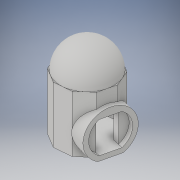
# Autodesk Inventor part: dome one terminal
Saved by Autodesk Inventor 2017 (Build 210142000, 142)
## iProperties
Created: 2018-03-05
Part Number: dome one terminal
Material: Generic
Document SubType Name: Modeling
Designer: Braxton
Density: 1 g/cm^3
Appearance: Default
Author: Braxton
Autodesk Inventor part; units mm, degrees
ref_plane "YZ Plane" through (0, 0, 0) normal (1, 0, 0) x (0, 1, 0)
ref_plane "XZ Plane" through (0, 0, 0) normal (0, 1, 0) x (-1, 0, 0)
ref_plane "XY Plane" through (0, 0, 0) normal (0, 0, 1) x (1, 0, 0)
sketch "Sketch1" plane through (0, 0, 0) normal (0, 1, 0) x (-1, 0, 0)
  line L0 (129.9296, -78.9016) -> (58.7381, -140.2035)
  line L1 (58.7381, -140.2035) -> (-34.8894, -147.9524)
  line L2 (-34.8894, -147.9524) -> (-115.1904, -99.1885)
  line L3 (-115.1904, -99.1885) -> (-151.4925, -12.538)
  line L4 (-151.4925, -12.538) -> (-129.9296, 78.9016)
  line L5 (-129.9296, 78.9016) -> (-58.7381, 140.2035)
  line L6 (-58.7381, 140.2035) -> (34.8894, 147.9524)
  line L7 (34.8894, 147.9524) -> (115.1904, 99.1885)
  line L8 (115.1904, 99.1885) -> (151.4925, 12.538)
  line L9 (151.4925, 12.538) -> (129.9296, -78.9016)
  point P0 (0, 0)
  point P1 (0, 0)
  dimension "d0" = 289.1411
  constraints: 20 end point, 1 coincident, 21 other
  measures "d0" distance between parallel lines of L5 L0
extrude "bace" add sketch "Sketch1" along normal blind 25.4
sketch "Sketch2" plane through (0, 25.4, 0) normal (0, 1, 0) x (1, 0, 0)
  line L0 (-58.7381, 140.2035) -> (-129.9296, 78.9016) projected
  line L1 (-129.9296, 78.9016) -> (-58.7381, 140.2035)
  line L2 (-58.7381, 140.2035) -> (34.8894, 147.9524)
  line L3 (34.8894, 147.9524) -> (115.1904, 99.1885)
  line L4 (115.1904, 99.1885) -> (151.4925, 12.538)
  line L5 (151.4925, 12.538) -> (129.9296, -78.9016)
  line L6 (129.9296, -78.9016) -> (58.7381, -140.2035)
  line L7 (58.7381, -140.2035) -> (-34.8894, -147.9524)
  line L8 (-34.8894, -147.9524) -> (-115.1904, -99.1885)
  line L9 (-115.1904, -99.1885) -> (-151.4925, -12.538)
  line L10 (-151.4925, -12.538) -> (-129.9296, 78.9016)
  line L11 (-107.1019, 65.0392) -> (-48.4182, 115.5708)
  line L12 (-48.4182, 115.5708) -> (28.7596, 121.9582)
  line L13 (28.7596, 121.9582) -> (94.9523, 81.7618)
  line L14 (94.9523, 81.7618) -> (124.8764, 10.3351)
  line L15 (124.8764, 10.3351) -> (107.1019, -65.0392)
  line L16 (107.1019, -65.0392) -> (48.4182, -115.5708)
  line L17 (48.4182, -115.5708) -> (-28.7596, -121.9582)
  line L18 (-28.7596, -121.9582) -> (-94.9523, -81.7618)
  line L19 (-94.9523, -81.7618) -> (-124.8764, -10.3351)
  line L20 (-124.8764, -10.3351) -> (-107.1019, 65.0392)
  line L21 (-129.9296, 78.9016) -> (-151.4925, -12.538) projected
  point P0 (0, 0)
  point P1 (0, 0)
  point P2 (0, 0)
  dimension "d4" = 25.4
  constraints: 40 end point, 2 coincident, 1 parallel, 42 other
  measures "d4" distance between parallel lines of L21 L20
extrude "bace wall" add sketch "Sketch2" along normal blind 254
sketch "Sketch3" plane through (0, 279.4, 0) normal (0, 1, 0) x (1, 0, 0)
  line L0 (-115.1904, -99.1885) -> (-151.4925, -12.538) projected
  circle A0 centre (0, 0) radius 119.1705
  line L1 (-58.7381, 140.2035) -> (-129.9296, 78.9016)
  line L2 (-129.9296, 78.9016) -> (-151.4925, -12.538)
  line L3 (-151.4925, -12.538) -> (-115.1904, -99.1885)
  line L4 (-115.1904, -99.1885) -> (-34.8894, -147.9524)
  line L5 (-34.8894, -147.9524) -> (58.7381, -140.2035)
  line L6 (58.7381, -140.2035) -> (129.9296, -78.9016)
  line L7 (129.9296, -78.9016) -> (151.4925, 12.538)
  line L8 (151.4925, 12.538) -> (115.1904, 99.1885)
  line L9 (115.1904, 99.1885) -> (34.8894, 147.9524)
  line L10 (34.8894, 147.9524) -> (-58.7381, 140.2035)
  line L11 (-129.9296, 78.9016) -> (-58.7381, 140.2035) projected
  line L12 (34.8894, 147.9524) -> (115.1904, 99.1885) projected
  line L13 (115.1904, 99.1885) -> (151.4925, 12.538) projected
  line L14 (151.4925, 12.538) -> (129.9296, -78.9016) projected
  line L15 (-34.8894, -147.9524) -> (58.7381, -140.2035) projected
  line L16 (-124.8764, -10.3351) -> (-107.1019, 65.0392) projected
  point P0 (-115.9892, 27.352)
  constraints: 20 end point, 2 coincident, 1 midpoint, 3 other
extrude "bace cieiling" add sketch "Sketch3" along normal blind 25.4
ref_plane "dome work plane" through (8.8872, 25.4, -37.6872) normal (0.9733039, 0, 0.22952) x (0.22952, 0, -0.9733039)
sketch "Sketch10" plane through (8.8872, 25.4, -37.6872) normal (0.9733039, 0, 0.22952) x (0.22952, 0, -0.9733039)
  line L0 (105.8497, 279.4) -> (80.4497, 279.4)
  line L1 (-157.8914, 279.4) -> (80.4497, 279.4) projected
  arc A0 (80.4497, 279.4) -> (-38.7209, 398.5705) centre (-38.7209, 279.4) ccw
  arc A1 (105.8497, 279.4) -> (-38.7209, 423.9705) centre (-38.7209, 279.4) ccw
  line L2 (-38.7209, 423.9705) -> (-38.7209, 398.5705)
  line L3 (-38.7209, 398.5705) -> (-38.7209, 279.4) construction
  point P0 (-38.7209, -25.4)
  dimension "d32" = 119.1705
  dimension "d33" = 144.5705
  constraints: 6 end point, 4 point on circle, 2 centre point, 2 coincident, 2 vertical, 1 midpoint
  measures "d32" radius of A0
  measures "d33" radius of A1
revolve "dome" add sketch "Sketch10" angle 360 about axis through (0, 423.9705, 0) along (0, -1, 0)
sketch "Sketch8" plane through (151.4925, 0, -12.538) normal (0.9733039, 0, 0.22952) x (0.22952, 0, -0.9733039)
  line L0 (-46.9738, 25.4) -> (3.8262, 25.4)
  line L1 (3.8262, 25.4) -> (3.8262, 194.7333)
  line L2 (3.8262, 194.7333) -> (-46.9738, 194.7333)
  line L3 (-46.9738, 194.7333) -> (-46.9738, 25.4)
  line L4 (-46.9738, 25.4) -> (-97.7738, 25.4)
  line L5 (-97.7738, 25.4) -> (-97.7738, 194.7333)
  line L6 (-97.7738, 194.7333) -> (-46.9738, 194.7333)
  line L7 (-85.6947, 25.4) -> (-8.253, 25.4) projected
  line L8 (-46.9738, 25.4) -> (-46.9738, 0) construction
  dimension "d16" = 50.8
  dimension "d17" = 169.3333
  constraints: 16 end point, 2 collinear, 2 symmetric about line, 1 horizontal, 1 midpoint, 1 perpendicular, 1 vertical
  measures "d16" distance of L0.start L0.end
  measures "d17" distance of L0.end L1.end
extrude "door frame" cut sketch "Sketch8" against normal blind 42.8625
sketch "Sketch7" plane through (151.4925, 0, -12.538) normal (0.9733039, 0, 0.22952) x (0.22952, 0, -0.9733039)
  line L0 (-97.7738, 194.7333) -> (3.8262, 194.7333)
  line L1 (-97.7738, 25.4) -> (3.8262, 25.4)
  arc A0 (10.4321, 0) -> (-104.3797, 0) centre (-46.9738, 110.0667) ccw
  arc A1 (-97.7738, 194.7333) -> (-97.7738, 25.4) centre (-46.9738, 110.0667) ccw
  arc A2 (3.8262, 25.4) -> (3.8262, 194.7333) centre (-46.9738, 110.0667) ccw
  line L2 (-104.3797, 0) -> (10.4321, 0)
  line L3 (-93.9476, 0) -> (-93.9476, 304.8) projected
  line L4 (-93.9476, 194.7333) -> (-93.9476, 224.9734)
  line L5 (-85.6947, 25.4) -> (-148.3463, 25.4) projected
  line L6 (-93.9476, 25.4) -> (-93.9476, 0)
  line L7 (0, 0) -> (0, 304.8) projected
  line L8 (0, 224.9734) -> (0, 194.7333)
  line L9 (0, 25.4) -> (0, 0)
  point P0 (-46.9738, 0)
  point P1 (-46.9738, 0)
  dimension "d14" = 169.3333
  dimension "d15" = 101.6
  dimension "d36" = 25.4
  dimension "d37" = 25.4
  constraints: 14 end point, 12 point on line, 8 point on circle, 3 centre point, 3 coincident, 2 horizontal, 2 parallel, 1 collinear, 1 concentric, 1 midpoint
  measures "d14" distance between parallel lines of L1 L0
  measures "d15" distance of L0.start L0.end
  measures "d36" distance between parallel lines of L2 L1
  measures "d37" radial gap between concentric circles of A0 A1
extrude "corridor connection" add sketch "Sketch7" along normal blind 25.4 contours A1 L5 A0 L3 L0 | L3 A0 L7 L0 | L1 L3 L2 A0 L5 | L7 A0 L2 L1 A2 L0 | L1 L7 L2 L3
sketch "Sketch11" plane through (151.4925, 224.9734, -12.538) normal (0.9733039, 0, 0.22952) x (0.22952, 0, -0.9733039)
  line L0 (76.0052, -224.9734) -> (0, -224.9734) projected
  line L1 (-85.6947, -30.2401) -> (-97.7738, -30.2401) projected
  line L2 (0, -224.9734) -> (0, 79.8266) projected
  line L3 (-93.9476, -30.2401) -> (-93.9476, 0)
  line L4 (0, 0) -> (0, -30.2401)
  line L5 (-93.9476, -224.9734) -> (0, -224.9734) projected
  line L6 (-93.9476, -224.9734) -> (-93.9476, -205.7351)
  line L7 (0, -208.7724) -> (0, -224.9734)
  line L8 (-104.3797, -224.9734) -> (-93.9476, -224.9734)
  line L9 (0, -224.9734) -> (10.4321, -224.9734)
  arc A0 (10.4321, -224.9734) -> (0, 0) centre (-46.9738, -114.9068) ccw
  arc A1 (-93.9476, 0) -> (-104.3797, -224.9734) centre (-46.9738, -114.9068) ccw
  line L10 (-97.7738, -30.2401) -> (-93.9476, -30.2401)
  line L11 (0, -30.2401) -> (3.8262, -30.2401)
  line L12 (-97.7738, -199.5734) -> (-93.9476, -199.5734)
  line L13 (-85.6947, -199.5734) -> (-148.3463, -199.5734) projected
  line L14 (-93.9476, -205.7351) -> (-93.9476, -199.5734)
  line L15 (0, -208.7724) -> (0, -199.5734)
  line L16 (3.8262, -199.5734) -> (0, -199.5734) projected
  line L17 (0, -199.5734) -> (3.8262, -199.5734)
  line L18 (-97.7738, -30.2401) -> (-97.7738, -199.5734) projected
  line L19 (-97.7738, -30.2401) -> (-97.7738, -199.5734)
  line L20 (3.8262, -30.2401) -> (3.8262, -199.5734) projected
  line L21 (3.8262, -30.2401) -> (3.8262, -199.5734)
  arc A2 (0, 0) -> (-93.9476, 0) centre (-46.9738, -114.9068) ccw projected
  arc A3 (-93.9476, 0) -> (-104.3797, -224.9734) centre (-46.9738, -114.9068) ccw projected
  point P0 (-46.9738, -224.9734)
  point P1 (-38.7209, -117.9441)
  point P2 (3.8262, -199.5734)
  constraints: 28 end point, 9 point on line, 4 collinear, 4 point on circle, 2 centre point, 2 concentric, 2 perpendicular, 1 horizontal alignment, 1 vertical
extrude "hide sliding doors" add sketch "Sketch11" against normal up to next contours L0 L2 L16 L20 L11 A0 | L8 A1 L13 L12 L14 L6 | L3 L1 L18 L13 A1
sketch "Sketch9" plane through (104.3295, 25.4, 76.7959) normal (0.22952, 0, -0.9733039) x (-0.9733039, 0, -0.22952)
  line L0 (-12.7, 169.3333) -> (-6.35, 169.3333)
  line L1 (-6.35, 169.3333) -> (-6.35, 0)
  line L2 (-6.35, 0) -> (-19.05, 0)
  line L3 (-19.05, 0) -> (-19.05, 169.3333)
  line L4 (-12.7, 169.3333) -> (-19.05, 169.3333)
  line L5 (-25.4, 199.5734) -> (-25.4, 208.8041) projected
  point P0 (119.1705, -25.4)
  point P1 (-25.4, -25.4)
  point P2 (-25.4, 169.3333)
  point P3 (0, 169.3333)
  point P4 (-25.4, 0)
  point P5 (0, 0)
  point P6 (-25.4, 169.3333)
  point P7 (-25.4, -25.1668)
  dimension "d22" = 6.35
  dimension "d23" = 12.7
  dimension "d24" = 169.3333
  constraints: 10 end point, 1 point on line
  measures "d22" distance of L0.start L0.end
  measures "d23" distance of L1.end L2.end
  measures "d24" distance between parallel lines of L2 L0
body "Solid1"
